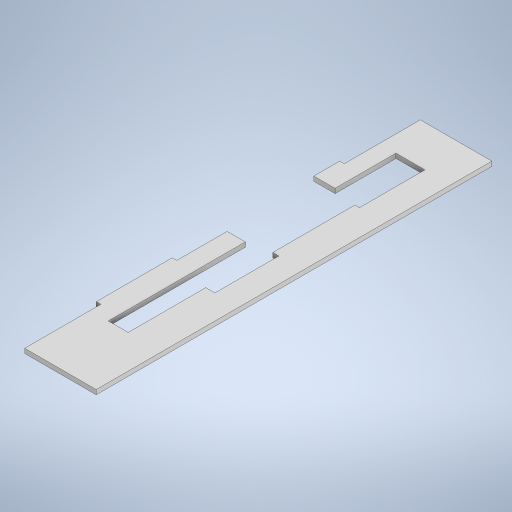
# Autodesk Inventor part: Atas Terminal
Saved by Autodesk Inventor 2024 (Build 280153000, 153)
## iProperties
Created: 2023-08-09
Part Number: Atas Terminal
Material: Generic
Document SubType Name: Modeling
Designer: Asus
Density: 1 g/cm^3
Appearance: Default
Author: Asus
Autodesk Inventor part; units mm, degrees
ref_plane "YZ Plane" through (0, 0, 0) normal (1, 0, 0) x (0, 1, 0)
ref_plane "XZ Plane" through (0, 0, 0) normal (0, 1, 0) x (-1, 0, 0)
ref_plane "XY Plane" through (0, 0, 0) normal (0, 0, 1) x (1, 0, 0)
sketch "Sketch1" plane through (0, 0, 0) normal (0, 1, 0) x (-1, 0, 0)
  line L0 (0, 0) -> (0, -260)
  line L1 (0, -260) -> (47, -260)
  line L2 (47, -260) -> (47, -210)
  line L3 (47, -210) -> (50, -210)
  line L4 (47, -100) -> (50, -100)
  line L5 (50, -100) -> (50, -50)
  line L6 (50, -50) -> (47, -50)
  line L7 (47, -50) -> (47, 0)
  line L8 (47, 0) -> (0, 0)
  line L9 (47, -260) -> (50, -260) construction
  line L10 (47, -100) -> (47, -133)
  line L11 (47, -260) -> (36, -260) construction
  line L12 (36, -233) -> (17, -233)
  line L13 (17, -233) -> (17, -190)
  line L14 (17, -190) -> (20, -190)
  line L15 (47, -133) -> (35, -133) construction
  line L16 (35, -133) -> (35, -43)
  line L17 (35, -43) -> (22, -43)
  line L18 (22, -43) -> (22, -94)
  line L19 (22, -94) -> (16, -94)
  line L20 (16, -94) -> (16, -136)
  line L21 (16, -136) -> (20, -136)
  line L22 (20, -190) -> (20, -136)
  line L23 (47, -133) -> (35, -133)
  line L24 (50, -210) -> (50, -193)
  line L25 (36, -193) -> (50, -193)
  line L26 (36, -193) -> (36, -233)
  dimension "d0" = 260
  dimension "d1" = 47
  dimension "d2" = 50
  dimension "d3" = 3
  dimension "d6" = 50
  dimension "d10" = 11
  dimension "d14" = 19
  dimension "d15" = 12
  dimension "d16" = 90
  dimension "d17" = 13
  dimension "d18" = 51
  dimension "d19" = 6
  dimension "d20" = 42
  dimension "d24" = 67
  dimension "d25" = 60
  constraints: 54 end point, 12 perpendicular, 4 vertical, 1 horizontal, 1 point on line
  measures "d0" distance of L0.start L0.end
  measures "d1" distance of L0.end L1.end
  measures "d2" distance of L1.end L2.end
  measures "d3" distance of L2.end L3.end
  measures "d6" distance of L4.end L5.end
  measures "d10" distance of L1.end L11.end
  measures "d14" distance of L12.start L12.end
  measures "d15" distance of L10.end L15.end
  measures "d16" distance of L15.end L16.end
  measures "d17" distance of L16.end L17.end
  measures "d18" distance of L17.end L18.end
  measures "d19" distance of L18.end L19.end
  measures "d20" distance of L19.end L20.end
  measures "d24" distance between parallel lines of L1 L25
  measures "d25" distance between parallel lines of L25 L23
extrude "Extrusion1" add sketch "Sketch1" along normal blind 3
body "Solid1"
